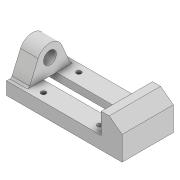
# Autodesk Inventor part: first
Saved by Autodesk Inventor 2020 (Build 240168000, 168)
## iProperties
Created: 2021-12-09
Part Number: first
Material: Generic
Document SubType Name: Modeling
Designer: NIKHIL VINOD
Density: 1 g/cm^3
Appearance: Default
Author: NIKHIL VINOD
Autodesk Inventor part; units mm, degrees
ref_plane "YZ Plane" through (0, 0, 0) normal (1, 0, 0) x (0, 1, 0)
ref_plane "XZ Plane" through (0, 0, 0) normal (0, 1, 0) x (-1, 0, 0)
ref_plane "XY Plane" through (0, 0, 0) normal (0, 0, 1) x (1, 0, 0)
sketch "Sketch1" plane through (0, 0, 0) normal (0, 0, 1) x (1, 0, 0)
  line L0 (12.9321, 0) -> (108.9321, 0)
  line L1 (108.9321, -16) -> (-9.0679, -16)
  line L2 (-9.0679, -16) -> (-9.0679, 0)
  line L3 (12.9321, 0) -> (12.9321, 36)
  line L4 (12.9321, 36) -> (-9.0679, 36)
  line L5 (-9.0679, 36) -> (-9.0679, 0)
  line L6 (108.9321, -16) -> (134.9321, -16)
  line L7 (134.9321, -16) -> (134.9321, 14)
  line L8 (108.9321, 0) -> (108.9321, 26)
  line L9 (108.9321, 26) -> (118.9321, 26)
  line L10 (118.9321, 26) -> (134.9321, 14)
  point P0 (0, 0)
  dimension "d0" = 118
  dimension "d1" = 16
  dimension "d2" = 22
  dimension "d3" = 36
  dimension "d4" = 26
  dimension "d5" = 30
  dimension "d6" = 26
  dimension "d7" = 10
  constraints: 22 end point, 2 horizontal, 2 parallel, 2 perpendicular, 1 vertical
  measures "d0" distance of L1.start L1.end
  measures "d1" distance of L0.end L1.start
  measures "d2" distance of L4.end L3.end
  measures "d3" distance of L0.start L3.end
  measures "d4" distance of L1.start L6.end
  measures "d5" distance of L6.end L7.end
  measures "d6" distance of L0.end L8.end
  measures "d7" distance of L8.end L9.end
extrude "Extrusion1" add sketch "Sketch1" along normal blind 64
sketch "Sketch2" plane through (-9.0679, -16, 0) normal (-1, 0, 0) x (0, 0, 1)
  circle A0 centre (32, 36) radius 8
  line L0 (0, 0) -> (64, 0) projected
  line L1 (0, 52) -> (0, 0) projected
  line L2 (0, 16) -> (64, 16) projected
  line L3 (0, 16) -> (4.0233, 16)
  line L4 (64, 16) -> (59.9767, 16)
  arc A1 (46.702, 42.3127) -> (17.298, 42.3127) centre (32, 36) ccw
  line L5 (57.2201, 17.8164) -> (46.702, 42.3127)
  line L6 (6.7799, 17.8164) -> (17.298, 42.3127)
  arc A2 (4.0233, 16) -> (6.7799, 17.8164) centre (4.0233, 19) ccw
  arc A3 (57.2201, 17.8164) -> (59.9767, 16) centre (59.9767, 19) ccw
  line L7 (0, 16) -> (0, 52)
  line L8 (0, 52) -> (64, 52) projected
  line L9 (64, 52) -> (64, 16)
  line L10 (64, 52) -> (64, 0) projected
  point P0 (6, 16)
  point P1 (58, 16)
  point P2 (32, 52)
  dimension "d10" = 16
  dimension "d11" = 36
  dimension "d12" = 32
  dimension "d13" = 6
  dimension "d14" = 6
  dimension "d15" = 3
  dimension "d16" = 3
  constraints: 12 end point, 6 point on circle, 6 point on line, 6 tangent, 4 centre point, 2 collinear, 1 coincident
  measures "d10" diameter of A0
  measures "d11" distance from line of L0 A0.centre
  measures "d12" distance from line of L1 A0.centre
  measures "d13" distance of L2.start point (6, 16)
  measures "d14" distance of L2.end point (58, 16)
  measures "d15" radius of A2
  measures "d16" radius of A3
extrude "Extrusion2" cut sketch "Sketch2" against normal blind 22 contours A0 | L1 L8 A1 L6 A2 L2 | L2 A3 L5 A1 L8 L9
sketch "Sketch3" plane through (-9.0679, -16, 0) normal (-1, 0, 0) x (0, 0, 1)
  line L0 (0, 0) -> (64, 0) projected
  line L1 (0, 16) -> (64, 16) projected
  line L2 (48, 0) -> (16, 0)
  line L3 (16, 0) -> (16, 7)
  line L4 (24, 16) -> (40, 16)
  line L5 (48, 7) -> (48, 0)
  line L6 (0, 16) -> (0, 0) projected
  line L7 (64, 16) -> (64, 0) projected
  line L8 (24, 16) -> (24, 7)
  line L9 (24, 7) -> (16, 7)
  line L10 (48, 7) -> (40, 7)
  line L11 (40, 7) -> (40, 16)
  point P0 (16, 0)
  dimension "d19" = 16
  dimension "d20" = 16
  dimension "d21" = 9
  dimension "d22" = 8
  dimension "d23" = 8
  constraints: 16 end point, 4 perpendicular, 3 parallel, 1 horizontal, 1 point on line
  measures "d19" distance between parallel lines of L6 L3
  measures "d20" distance between parallel lines of L7 L5
  measures "d21" distance of L4.start L8.end
  measures "d22" distance of L5.start L10.end
  measures "d23" distance of L3.end L8.end
extrude "Extrusion3" cut sketch "Sketch3" against normal blind 118 contours L3 L9 L8 L1 L11 L10 L5 L0
sketch "Sketch4" plane through (-9.0679, -16, 0) normal (0, -1, 0) x (1, 0, 0)
  circle A0 centre (36, 54) radius 3
  line L0 (0, 48) -> (0, 64) projected
  line L1 (0, 64) -> (144, 64) projected
  circle A1 centre (106, 54) radius 3
  circle A2 centre (36, 10) radius 3
  circle A3 centre (106, 10) radius 3
  point P0 (9.0679, 0)
  dimension "d26" = 6
  dimension "d27" = 36
  dimension "d28" = 10
  dimension "d31" = 70
  dimension "d34" = 44
  constraints: 4 centre point, 1 horizontal, 1 vertical, 6 other
  measures "d26" diameter of A0
  measures "d27" distance from line of A0.centre L0
  measures "d28" distance from line of L1 A0.centre
  measures "d31" distance of A0.centre A1.centre
  measures "d34" distance of A0.centre A2.centre
extrude "Extrusion4" cut sketch "Sketch4" against normal through all
body "Solid1"
